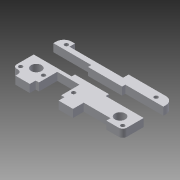
# Autodesk Inventor part: XcrRight_b
Saved by Autodesk Inventor 2013 (Build 170138000, 138)
## iProperties
Created: 2015-01-14
Part Number: XcrRight_b
Material: Generic
Document SubType Name: Modeling
Designer: dzban
Density: 1 g/cm^3
Author: dzban
Autodesk Inventor part; units mm, degrees
ref_plane "YZ Plane" through (0, 0, 0) normal (1, 0, 0) x (0, 1, 0)
ref_plane "XZ Plane" through (0, 0, 0) normal (0, 1, 0) x (-1, 0, 0)
ref_plane "XY Plane" through (0, 0, 0) normal (0, 0, 1) x (1, 0, 0)
sketch "Sketch1" plane through (0, 0, 0) normal (0, 0, 1) x (1, 0, 0)
  arc A0 (26.3204, -8.0097) -> (29.3204, -5.0097) centre (26.3204, -5.0097) ccw
  line L0 (29.3204, 7.9903) -> (29.3204, -5.0097)
  line L1 (0.3204, 7.9903) -> (29.3204, 7.9903)
  line L2 (0.3204, 10.4903) -> (0.3204, 7.9903)
  line L3 (-25.6796, 10.4903) -> (0.3204, 10.4903)
  line L4 (-25.6796, 7.9903) -> (-25.6796, 10.4903)
  line L5 (-54.6796, 7.9903) -> (-25.6796, 7.9903)
  line L6 (-54.6796, -5.0097) -> (-54.6796, 7.9903)
  arc A1 (-54.6796, -5.0097) -> (-51.6796, -8.0097) centre (-51.6796, -5.0097) ccw
  line L7 (-50.6796, -8.0097) -> (-51.6796, -8.0097)
  arc A2 (-47.6796, -11.0097) -> (-50.6796, -8.0097) centre (-50.6796, -11.0097) ccw
  line L8 (-47.6796, -13.0097) -> (-47.6796, -11.0097)
  line L9 (-36.6796, -13.0097) -> (-47.6796, -13.0097)
  line L10 (-36.6796, -8.5097) -> (-36.6796, -13.0097)
  line L11 (-34.1796, -8.5097) -> (-36.6796, -8.5097)
  line L12 (-34.1796, 5.4903) -> (-34.1796, -8.5097)
  line L13 (-17.1796, 5.4903) -> (-34.1796, 5.4903)
  line L14 (-17.1796, -8.5097) -> (-17.1796, 5.4903)
  line L15 (-14.6796, -8.5097) -> (-17.1796, -8.5097)
  line L16 (-14.6796, -13.0097) -> (-14.6796, -8.5097)
  line L17 (-3.6796, -13.0097) -> (-14.6796, -13.0097)
  line L18 (-3.6796, -4.8097) -> (-3.6796, -13.0097)
  line L19 (16.8204, -4.8097) -> (-3.6796, -4.8097)
  line L20 (16.8204, -8.0097) -> (16.8204, -4.8097)
  line L21 (26.3204, -8.0097) -> (16.8204, -8.0097)
  circle A3 centre (-44.6796, -0.0097) radius 3.96
  circle A4 centre (19.3204, -0.0097) radius 3.96
  circle A5 centre (-37.1796, -2.0097) radius 1.5
  circle A6 centre (-14.1796, -2.0097) radius 1.5
  circle A7 centre (-51.6796, -5.0097) radius 1.5
  circle A8 centre (26.3204, -5.0097) radius 1.5
  circle A9 centre (20.3204, 26.4903) radius 1.5
  circle A10 centre (-48.6796, 26.9903) radius 1.5
  arc A11 (-48.6796, 30.9903) -> (-54.6796, 24.9903) centre (-48.6796, 24.9903) ccw
  line L22 (-54.6796, 24.9903) -> (-54.6796, 22.9903)
  line L23 (-54.6796, 22.9903) -> (-25.6796, 22.9903)
  line L24 (-25.6796, 22.9903) -> (-25.6796, 20.4903)
  line L25 (-25.6796, 20.4903) -> (0.3204, 20.4903)
  line L26 (0.3204, 20.4903) -> (0.3204, 22.9903)
  line L27 (0.3204, 22.9903) -> (29.3204, 22.9903)
  line L28 (29.3204, 22.9903) -> (29.3204, 24.9903)
  arc A12 (29.3204, 24.9903) -> (23.3204, 30.9903) centre (23.3204, 24.9903) ccw
  line L29 (23.3204, 30.9903) -> (-5.1796, 30.9903)
  line L30 (-5.1796, 30.9903) -> (-5.1796, 26.7903)
  line L31 (-5.1796, 26.7903) -> (-46.1796, 26.7903)
  line L32 (-46.1796, 26.7903) -> (-46.1796, 30.9903)
  line L33 (-46.1796, 30.9903) -> (-48.6796, 30.9903)
  point P0 (0, 0)
  point P1 (0, 0)
  constraints: 68 end point, 13 centre point, 10 point on circle
extrude "Extrusion1" add sketch "Sketch1" along normal blind 6
body "Solid1"
